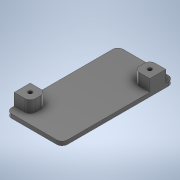
# Autodesk Inventor part: DCDC_Holder
Saved by Autodesk Inventor 2020 (Build 240168000, 168)
## iProperties
Created: 2020-04-25
Part Number: DCDC_Holder
Material: Типовые
Document SubType Name: Modeling
Designer: Михаил
Density: 1 g/cm^3
Appearance: По умолчанию
Author: Михаил
Autodesk Inventor part; units mm, degrees
ref_plane "YZ Plane" through (0, 0, 0) normal (1, 0, 0) x (0, 1, 0)
ref_plane "XZ Plane" through (0, 0, 0) normal (0, 1, 0) x (-1, 0, 0)
ref_plane "XY Plane" through (0, 0, 0) normal (0, 0, 1) x (1, 0, 0)
sketch "Эскиз1" plane through (0, 0, 0) normal (0, 1, 0) x (-1, 0, 0)
  line L0 (0, 0) -> (21, 0)
  line L1 (21, 0) -> (21, -42)
  line L2 (21, -42) -> (0, -42)
  line L3 (0, -42) -> (0, 0)
  dimension "d0" = 21
  dimension "d1" = 42
  constraints: 8 end point, 2 parallel, 1 horizontal, 1 perpendicular
  measures "d0" distance of L1.end L2.end
  measures "d1" distance of L0.end L1.end
extrude "Выдавливание1" add sketch "Эскиз1" along normal blind 1.5
sketch "Эскиз2" plane through (0, 1.5, 0) normal (0, 1, 0) x (1, 0, 0)
  line L0 (0, 0) -> (0, 42) projected
  line L1 (0, 39) -> (-6, 39)
  line L2 (-6, 39) -> (-6, 33)
  line L3 (-6, 33) -> (0, 33)
  line L4 (0, 33) -> (0, 39)
  line L5 (0, 42) -> (-21, 42) projected
  line L6 (-21, 42) -> (-21, 0) projected
  line L7 (-21, 3) -> (-15, 3)
  line L8 (-15, 3) -> (-15, 9)
  line L9 (-15, 9) -> (-21, 9)
  line L10 (-21, 9) -> (-21, 3)
  line L11 (-21, 0) -> (0, 0) projected
  point P0 (0, 33)
  dimension "d4" = 6
  dimension "d5" = 6
  dimension "d6" = 3
  dimension "d7" = 6
  dimension "d8" = 6
  dimension "d9" = 3
  constraints: 16 end point, 4 parallel, 2 horizontal, 2 perpendicular, 2 point on line
  measures "d4" distance of L3.end L2.end
  measures "d5" distance of L2.end L1.end
  measures "d6" distance between parallel lines of L5 L1
  measures "d7" distance of L9.end L8.end
  measures "d8" distance of L8.end L7.end
  measures "d9" distance between parallel lines of L11 L7
extrude "Выдавливание2" add sketch "Эскиз2" along normal blind 4.5 contours L3 L2 L1 L0 | L6 L9 L8 L7
fillet "Сопряжение1" radius 2 8 edges at (-15, 3.75, -3) (-15, 3.75, -9) (-6, 3.75, -33) (-6, 3.75, -39) (0, 0.75, 0) (0, 0.75, -42) (-21, 0.75, 0) (-21, 0.75, -42)
sketch "Эскиз3" plane through (0, 6, 0) normal (0, 1, 0) x (1, 0, 0)
  circle A0 centre (-18, 6) radius 0.75
  line L0 (-21, 9) -> (-21, 3) projected
  line L1 (-17, 9) -> (-21, 9) projected
  circle A1 centre (-3, 36) radius 0.75
  line L2 (0, 39) -> (-4, 39) projected
  line L3 (0, 33) -> (0, 39) projected
  point P0 (0, 0)
  dimension "d13" = 1.5
  dimension "d14" = 3
  dimension "d15" = 3
  dimension "d16" = 1.5
  dimension "d17" = 3
  dimension "d18" = 3
  constraints: 2 centre point
  measures "d13" diameter of A0
  measures "d14" distance from line of L0 A0.centre
  measures "d15" distance from line of L1 A0.centre
  measures "d16" diameter of A1
  measures "d17" distance from line of L2 A1.centre
  measures "d18" distance from line of L3 A1.centre
extrude "Выдавливание3" cut sketch "Эскиз3" against normal blind 5
